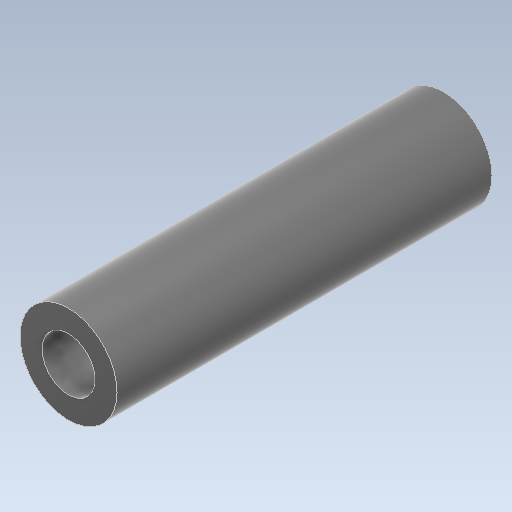
# Autodesk Inventor part: Pino_Pistão
Saved by Autodesk Inventor 2021 (Build 250183000, 183)
## iProperties
Created: 2021-07-11
Part Number: Pino_Pistão
Material: Genérico
Document SubType Name: Modeling
Designer: Giovanni
Density: 1 g/cm^3
Appearance: Liso - Preto
Author: Giovanni
Autodesk Inventor part; units mm, degrees
ref_plane "YZ Plane" through (0, 0, 0) normal (1, 0, 0) x (0, 1, 0)
ref_plane "XZ Plane" through (0, 0, 0) normal (0, 1, 0) x (-1, 0, 0)
ref_plane "XY Plane" through (0, 0, 0) normal (0, 0, 1) x (1, 0, 0)
sketch "Esboço2" plane through (0, 0, 0) normal (0, 0, 1) x (1, 0, 0)
  circle A0 centre (0, 0) radius 6
  circle A1 centre (0, 0) radius 11
  dimension "d4" = 12
  dimension "d5" = 22
  constraints: 2 centre point, 2 coincident
  measures "d4" diameter of A0
  measures "d5" diameter of A1
extrude "Extrusão2" add sketch "Esboço2" along normal mid plane 85
